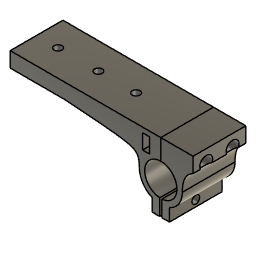
y-bearing-holder (Autodesk Fusion 360 design; units mm, degrees)
Autodesk Fusion 360 part; units mm, degrees
note: some values were not read from the file. Set by a fixed rule: which sketch regions a step uses.
sketch "front" plane through (0, 0, 0) normal (0, 1, 0) x (1, 0, 0) in component "bearing-holder"
  circle A0 centre (0, 0) radius 7.5
  line L0 (0, 0) -> (0, -15) construction
  line L1 (0, -15) -> (-70, -15)
  line L2 (-70, -15) -> (-70, 15)
  line L3 (-70, 15) -> (0, 15)
  line L4 (0, 15) -> (0, -15)
  line L5 (-70, -15) -> (0, -15)
  line L6 (0, -15) -> (0, -10)
  line L7 (0, -10) -> (-70, -10)
  line L8 (-70, -10) -> (-70, -15)
  circle A1 centre (0, 0) radius 10
  line L9 (-35, -10) -> (-45, -10) construction
  line L10 (0, 0) -> (-10, 0) construction
  line L11 (-10, 0) -> (-10, -7.5) construction
  spline S0 degree 2 poles (-10, 0) (-10, -7.5) (-45, -10) knots 0 0 0 3.893303 3.893303 3.893303 weights 1 3 1
  line L12 (0, 0) -> (-4, 0) construction
  line L13 (-4, 0) -> (-4, 15) construction
  line L14 (-4, 15) -> (0, 15) construction
  line L15 (0, 15) -> (0, 0) construction
  line L16 (0, 0) -> (-0.5, 0) construction
  line L17 (-0.5, 0) -> (-0.5, 15) construction
  line L18 (-0.5, 15) -> (0, 15) construction
  line L19 (0, 15) -> (0, 0) construction
  line L20 (-4, 6.3443) -> (-0.5, 6.3443)
  line L21 (-0.5, 6.3443) -> (-0.5, 15)
  line L22 (-0.5, 15) -> (-4, 15)
  line L23 (-4, 15) -> (-4, 6.3443)
  line L24 (0, -15) -> (15, -15)
  line L25 (15, -15) -> (15, 15)
  line L26 (15, 15) -> (0, 15)
  line L27 (0, 15) -> (0, -15)
  line L28 (0, 0) -> (0.5, 0) construction
  line L29 (0, 0) -> (4, 0) construction
  line L30 (0.5, 0) -> (4, 0) construction
  line L31 (4, 0) -> (4, 15) construction
  line L32 (4, 15) -> (0.5, 15) construction
  line L33 (0.5, 15) -> (0.5, 0) construction
  line L34 (4, 6.3443) -> (0.5, 6.3443)
  line L35 (0.5, 6.3443) -> (0.5, 15)
  line L36 (0.5, 15) -> (4, 15)
  line L37 (4, 15) -> (4, 6.3443)
  line L38 (0, -10) -> (15, -10) construction
  line L39 (0, 0) -> (10, 0) construction
  line L40 (10, 0) -> (10, -7.5) construction
  spline S1 degree 2 poles (10, 0) (10, -7.5) (15, -10) knots 0 0 0 1.167708 1.167708 1.167708
  dimension "d1" = 15
  dimension "d2" = 15
  dimension "d3" = 70
  dimension "d4" = 30
  dimension "d5" = 70
  dimension "d6" = 5
  dimension "d7" = 20
  dimension "d8" = 10
  dimension "d9" = 7.5
  dimension "d11" = 4
  dimension "d12" = 15
  dimension "d13" = 0.5
  dimension "d16" = 15
  dimension "d17" = 30
  dimension "d18" = 0.5
  dimension "d19" = 4
  dimension "d20" = 7.5
  constraint coincident A0.centre L0.start
  constraint vertical L0
  constraint horizontal L1
  constraint vertical L2
  constraint horizontal L3
  constraint vertical L4
  constraint horizontal L5
  constraint vertical L6
  constraint horizontal L7
  constraint vertical L8
  constraint concentric A0 A1
  constraint midpoint L7 L9.start
  constraint parallel L7 L9
  constraint coincident A1 L10.end
  constraint perpendicular L0 L10
  constraint perpendicular L10 L11
  constraint horizontal L12
  constraint vertical L13
  constraint horizontal L14
  constraint vertical L15
  constraint horizontal L16
  constraint vertical L17
  constraint horizontal L18
  constraint vertical L19
  constraint horizontal L20
  constraint vertical L21
  constraint horizontal L22
  constraint vertical L23
  constraint coincident L13 L20.start
  constraint coincident A0 L20.start
  constraint horizontal L24
  constraint vertical L25
  constraint horizontal L26
  constraint vertical L27
  constraint perpendicular L19 L28
  constraint parallel L28 L29
  constraint horizontal L30
  constraint vertical L31
  constraint horizontal L32
  constraint vertical L33
  constraint coincident L26 L31.end
  constraint horizontal L34
  constraint vertical L35
  constraint horizontal L36
  constraint vertical L37
  constraint coincident A0 L34.start
  constraint coincident L31 L34.start
  constraint coincident L25 L38.end
  constraint tangent A1 L38
  constraint perpendicular L25 L38
  constraint coincident A1 L39.end
  constraint parallel L30 L39
  constraint perpendicular L39 L40
  measures "d1" diameter of A0
  measures "d2" distance of A0.centre L0.end
  measures "d3" distance of L0.end L1.end
  measures "d4" distance of L0.end L3.end
  measures "d5" distance of L1.end L0.end
  measures "d6" distance of L1.end L7.end
  measures "d7" diameter of A1
  measures "d8" distance of L9.start L9.end
  measures "d9" distance of L10.end L11.end
  measures "d11" distance of A0.centre L12.end
  measures "d12" distance of A0.centre L3.end
  measures "d13" distance of A0.centre L16.end
  measures "d16" distance of L0.end L24.end
  measures "d17" distance of L0.end L3.end
  measures "d18" distance of A0.centre L28.end
  measures "d19" distance of A0.centre L29.end
  measures "d20" distance of L39.end L40.end
extrude "Extrude1" add sketch "front" along normal blind 24.5 contours A0 L4 A1 L23 L27 | A0 A1 L21 L23 | L1 L2 L4 L5 L6 L7 L8 L27 | L7 A1 S0 | L3 A1 L21 L22 L23 makes body 1 in component "bearing-holder"
extrude "Extrude2" add sketch "front" along normal blind 24.5 separate body contours A0 L4 A1 L27 L37 | A0 A1 L35 L37 | A1 L26 L35 L36 L37 | L4 L6 A1 L24 L25 L27 S1 makes body 2 in component "bearing-holder"
sketch "bottom-screws" plane through (4, 0, 0) normal (1, 0, 0) x (0, 1, 0) in component "bearing-holder"
  line L0 (0, -9.1652) -> (0, -15)
  line L1 (0, -15) -> (24.5, -15)
  line L2 (24.5, -15) -> (24.5, -9.1652)
  line L3 (24.5, -9.1652) -> (0, -9.1652)
  line L4 (0, -9.1652) -> (24.5, -15) construction
  line L5 (24.5, -9.1652) -> (0, -15) construction
  line L6 (12.25, -9.1652) -> (12.25, -15) construction
  line L7 (0, -9.1652) -> (12.25, -15) construction
  line L8 (12.25, -9.1652) -> (0, -15) construction
  line L9 (12.25, -9.1652) -> (24.5, -15) construction
  line L10 (24.5, -9.1652) -> (12.25, -15) construction
  circle A0 centre (6.125, -12.0826) radius 1.8
  circle A1 centre (18.375, -12.0826) radius 1.8
  circle A2 centre (12.25, -12.0826) radius 1.8
  dimension "d24" = 3.6
  dimension "d25" = 3.6
  dimension "d57" = 3.6
  constraint coincident L0.start L3.end
  constraint coincident L1.end L2.start
  constraint coincident L2.end L3.start
  constraint coincident L0.end L1.start
  constraint midpoint L3 L6.start
  constraint midpoint L1 L6.end
  constraint midpoint L8 A0.centre
  constraint midpoint L9 A1.centre
  constraint midpoint L6 A2.centre
  measures "d24" diameter of A0
  measures "d25" diameter of A1
  measures "d57" diameter of A2
sketch "upper-screws" plane through (0, 0, 0) normal (-1, 0, 0) x (0, -1, 0) in component "bearing-holder"
  line L0 (0, 7.5) -> (0, 15)
  line L1 (0, 15) -> (-24.5, 15)
  line L2 (-24.5, 15) -> (-24.5, 7.5)
  line L3 (-24.5, 7.5) -> (0, 7.5)
  line L4 (-24.5, 15) -> (0, 7.5) construction
  line L5 (0, 15) -> (-24.5, 7.5) construction
  line L6 (-12.25, 15) -> (-12.25, 7.5) construction
  line L7 (-24.5, 15) -> (-12.25, 7.5) construction
  line L8 (-12.25, 15) -> (-24.5, 7.5) construction
  line L9 (-12.25, 15) -> (0, 7.5) construction
  line L10 (0, 15) -> (-12.25, 7.5) construction
  circle A0 centre (-18.375, 11.25) radius 3
  circle A1 centre (-6.125, 11.25) radius 3
  circle A2 centre (-18.375, 11.25) radius 1.8
  circle A3 centre (-6.125, 11.25) radius 1.8
  line L11 (-15.375, 12.9821) -> (-18.375, 14.7141)
  line L12 (-18.375, 14.7141) -> (-21.375, 12.9821)
  line L13 (-21.375, 12.9821) -> (-21.375, 9.5179)
  line L14 (-21.375, 9.5179) -> (-18.375, 7.7859)
  line L15 (-18.375, 7.7859) -> (-15.375, 9.5179)
  line L16 (-15.375, 9.5179) -> (-15.375, 12.9821)
  line L17 (-9.125, 9.5179) -> (-6.125, 7.7859)
  line L18 (-6.125, 7.7859) -> (-3.125, 9.5179)
  line L19 (-3.125, 9.5179) -> (-3.125, 12.9821)
  line L20 (-3.125, 12.9821) -> (-6.125, 14.7141)
  line L21 (-6.125, 14.7141) -> (-9.125, 12.9821)
  line L22 (-9.125, 12.9821) -> (-9.125, 9.5179)
  line L23 (-18.375, 14.7141) -> (-24.5, 14.7141)
  line L24 (-24.5, 14.7141) -> (-24.5, 7.7859)
  line L25 (-24.5, 7.7859) -> (-18.375, 7.7859)
  line L26 (-18.375, 7.7859) -> (-18.375, 14.7141)
  line L27 (-6.125, 14.7141) -> (0, 14.7141)
  line L28 (0, 14.7141) -> (0, 7.7859)
  line L29 (0, 7.7859) -> (-6.125, 7.7859)
  line L30 (-6.125, 7.7859) -> (-6.125, 14.7141)
  point P0 (-18.375, 11.25)
  point P1 (-6.125, 11.25)
  dimension "d28" = 6
  dimension "d29" = 6
  dimension "d30" = 3.6
  dimension "d31" = 3.6
  dimension "d52" = 3
  dimension "d53" = 3
  constraint coincident L1.end L2.start
  constraint coincident L0.start L3.end
  constraint coincident L0.end L1.start
  constraint coincident L2.end L3.start
  constraint midpoint L1 L6.start
  constraint midpoint L3 L6.end
  constraint midpoint L8 P0
  constraint midpoint L10 P1
  constraint concentric A0 A2
  constraint concentric A1 A3
  constraint coincident P0 A0.centre
  constraint coincident P1 A1.centre
  constraint horizontal L23
  constraint vertical L24
  constraint horizontal L25
  constraint vertical L26
  constraint coincident L2 L24.end
  constraint horizontal L27
  constraint vertical L28
  constraint horizontal L29
  constraint vertical L30
  constraint coincident L0 L28.end
  constraint coincident L17.end L18.start
  constraint coincident L14.end L15.start
  measures "d28" diameter of A0
  measures "d29" diameter of A1
  measures "d30" diameter of A2
  measures "d31" diameter of A3
  measures "d52" distance of P0 L16
  measures "d53" distance of P1 L22
extrude "Extrude4" cut sketch "upper-screws" against normal blind 10 from surface at -5 contours A1 A3 L30 | A1 A3 L30 | A3 L30 | A3 L30 | A0 A2 L26 | A0 A2 L26 | A2 L26 | A2 L26 bodies 2 in component "bearing-holder"
extrude "Extrude5" cut sketch "upper-screws" along normal blind 11 and the other way blind 7.5 contours A3 L30 | A3 L30 | A2 L26 | A2 L26 bodies 1 2 in component "bearing-holder"
sketch "plate-mount" plane through (0, 0, 15) normal (0, 0, 1) x (-1, 0, 0) in component "bearing-holder"
  line L0 (70, 0) -> (0, 0)
  line L1 (0, 0) -> (0, -24.5)
  line L2 (0, -24.5) -> (70, -24.5)
  line L3 (70, -24.5) -> (70, 0)
  line L4 (70, -24.5) -> (60, -24.5) construction
  line L5 (60, -24.5) -> (60, 0) construction
  line L6 (60, 0) -> (70, 0) construction
  line L7 (70, 0) -> (70, -24.5) construction
  circle A0 centre (60, -12.25) radius 1.8
  line L8 (60, -24.5) -> (50, -24.5) construction
  line L9 (50, -24.5) -> (15, -24.5) construction
  line L10 (15, -24.5) -> (15, 0) construction
  line L11 (15, 0) -> (50, 0) construction
  line L12 (50, 0) -> (50, -24.5) construction
  line L13 (50, -24.5) -> (32.5, 0) construction
  line L14 (32.5, -24.5) -> (50, 0) construction
  line L15 (32.5, -24.5) -> (15, 0) construction
  line L16 (15, -24.5) -> (32.5, 0) construction
  circle A1 centre (41.25, -12.25) radius 1.8
  circle A2 centre (23.75, -12.25) radius 1.8
  circle A3 centre (41.25, -12.25) radius 3.1
  circle A4 centre (23.75, -12.25) radius 3.1
  dimension "d39" = 10
  dimension "d40" = 3.6
  dimension "d41" = 10
  dimension "d42" = 35
  dimension "d43" = 3.6
  dimension "d44" = 3.6
  dimension "d47" = 6.2
  dimension "d48" = 6.2
  constraint horizontal L4
  constraint vertical L5
  constraint horizontal L6
  constraint vertical L7
  constraint coincident L2.end L3.start
  constraint midpoint L5 A0.centre
  constraint coincident L2 L8.end
  constraint horizontal L9
  constraint vertical L10
  constraint horizontal L11
  constraint vertical L12
  constraint midpoint L11 L13.end
  constraint midpoint L9 L14.start
  constraint midpoint L13 A1.centre
  constraint midpoint L15 A2.centre
  constraint concentric A1 A3
  constraint concentric A2 A4
  measures "d39" distance of L2.end L4.end
  measures "d40" diameter of A0
  measures "d41" distance of L4.end L8.end
  measures "d42" distance of L8.end L9.end
  measures "d43" diameter of A1
  measures "d44" diameter of A2
  measures "d47" diameter of A3
  measures "d48" diameter of A4
extrude "Extrude6" cut sketch "plate-mount" against normal blind 7 contours A0 | A1 | A2 bodies 1 in component "bearing-holder"
extrude "Extrude7" cut sketch "plate-mount" along normal blind 2 from surface at -7 contours A3 | A4 bodies 1 in component "bearing-holder"
extrude "Extrude8" cut sketch "upper-screws" along normal blind 3.2 from surface at 5.25 contours L0 L18 L19 L20 L27 L28 L29 | A1 L18 L30 | A1 L17 L30 | L2 L12 L13 L14 L23 L24 L25 | A1 L21 L30 | A1 L20 L30 | A1 L17 L22 | A1 A3 L30 | A1 A3 L30 | A1 L18 L19 | A0 L15 L26 | A0 L14 L26 | A1 L19 L20 | A1 L21 L22 | A0 L12 L26 | A0 L11 L26 | A0 L13 L14 | A0 A2 L26 | A0 A2 L26 | A0 L15 L16 | A0 L11 L16 | A0 L12 L13 bodies 1 in component "bearing-holder"
extrude "Extrude9" cut sketch "bottom-screws" against normal blind 8 contours A2 bodies 1 2 in component "bearing-holder"
extrude "Extrude10" add 1 faces at (5, 8.1667, 15) along direction (0, 0, 1) blind 2 on bodies 2 bodies 2 in component "bearing-holder"
extrude "Extrude11" add 1 faces at (-7.3167, 12.25, 15) along direction (0, 0, 1) blind 2 on bodies 1 bodies 1 in component "bearing-holder"
delete_face "DeleteFace1" 1 faces at (-20.8872, 12.5465, 8) on bodies 1 in component "bearing-holder"
component "bearing-holder" placed x (1, 0, 0) y (0, 1, 0) z (0, 0, 1) at (0, 0, 0)
equation "d42 = 50 mm - 15 mm"
equation "d54 = ( ( 7.5 / 2 ) * 1 mm ) + 1.5 mm"
named bodies: "outer", "inner"
